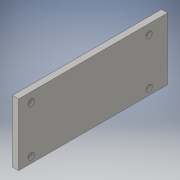
# Autodesk Inventor part: sideplate
Saved by Autodesk Inventor 2016 (Build 200138000, 138)
## iProperties
Created: 2017-01-05
Part Number: sideplate
Material: Generic
Document SubType Name: Modeling
Designer: james
Density: 1 g/cm^3
Appearance: Default
Author: james
Autodesk Inventor part; units mm, degrees
ref_plane "YZ Plane" through (0, 0, 0) normal (1, 0, 0) x (0, 1, 0)
ref_plane "XZ Plane" through (0, 0, 0) normal (0, 1, 0) x (-1, 0, 0)
ref_plane "XY Plane" through (0, 0, 0) normal (0, 0, 1) x (1, 0, 0)
sketch "Sketch1" plane through (0, 0, 0) normal (1, 0, 0) x (0, 1, 0)
  line L0 (22.1374, 30.7428) -> (-3.2626, 30.7428)
  line L1 (-3.2626, 30.7428) -> (-3.2626, -30.2172)
  line L2 (-3.2626, -30.2172) -> (22.1374, -30.2172)
  line L3 (22.1374, -30.2172) -> (22.1374, 30.7428)
  point P0 (0, 0)
  dimension "d0" = 60.96
  dimension "d1" = 25.4
  constraints: 8 end point, 2 parallel, 1 horizontal, 1 perpendicular
  measures "d0" distance of L2.end L0.start
  measures "d1" distance of L0.start L0.end
extrude "Extrusion1" add sketch "Sketch1" along normal blind 2.54
sketch "Sketch2" plane through (2.54, 0, 0) normal (1, 0, 0) x (0, 0, -1)
  line L0 (-30.7428, -3.2626) -> (30.2172, -3.2626) projected
  point P0 (0, 0)
  point P1 (-25.6628, 18.3274)
  point P2 (-25.6628, -0.7226)
  point P3 (22.5972, -0.7226)
  point P4 (22.5972, 18.3274)
  dimension "d4" = 0
  dimension "d5" = 0
  dimension "d6" = 0
  dimension "d7" = 0
  dimension "d8" = 19.05
  dimension "d9" = 2.54
  dimension "d10" = 5.08
  dimension "d11" = 48.26
  measures "d4" horizontal distance of point (-25.663, -0.723) point (-25.663, 18.327)
  measures "d5" vertical distance of point (22.597, -0.723) point (-25.663, -0.723)
  measures "d6" horizontal distance of point (22.597, 18.327) point (22.597, -0.723)
  measures "d7" vertical distance of point (-25.663, 18.327) point (22.597, 18.327)
  measures "d8" distance of point (-25.663, -0.723) point (-25.663, 18.327)
  measures "d9" distance from line of L0 point (-25.663, -0.723)
  measures "d10" horizontal distance of point (-25.663, 18.327) L0.start
  measures "d11" distance of point (-25.663, 18.327) point (22.597, 18.327)
hole "Hole1" at (2.54, 18.3274, 25.6628) at (2.54, -0.7226, 25.6628) at (2.54, -0.7226, -22.5972) at (2.54, 18.3274, -22.5972) direction (-1, 0, 0) diameter 2.54 end through all
body "Solid1"
